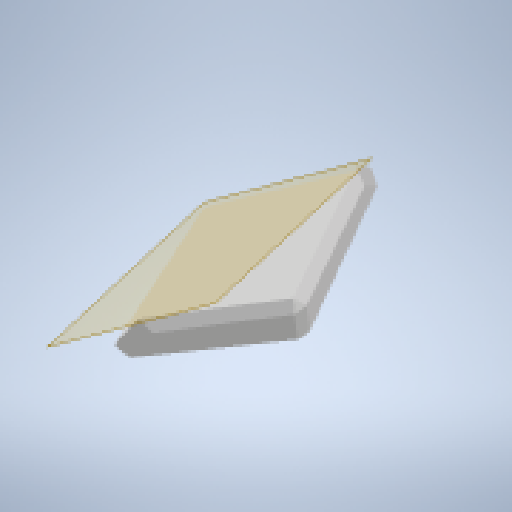
# Autodesk Inventor part: Union
Saved by Autodesk Inventor 2024 (Build 280153000, 153)
## iProperties
Created: 2024-04-21
Part Number: Union
Material: Genérico
Document SubType Name: Modeling
Designer: sergi
Density: 1 g/cm^3
Appearance: Valor por defecto
Author: sergi
Autodesk Inventor part; units mm, degrees
ref_plane "YZ Plane" through (0, 0, 0) normal (1, 0, 0) x (0, 1, 0)
ref_plane "XZ Plane" through (0, 0, 0) normal (0, 1, 0) x (-1, 0, 0)
ref_plane "XY Plane" through (0, 0, 0) normal (0, 0, 1) x (1, 0, 0)
ref_plane "Plano de trabajo1" through (154.464, -212.6015, -162.4131) normal (0.8506508, -0.2763932, -0.4472136) x (0.5, 0.688191, 0.5257311)
sketch "Boceto1" plane through (154.464, -212.6015, -162.4131) normal (0.8506508, -0.2763932, -0.4472136) x (0.5, 0.688191, 0.5257311)
  line L0 (7.992, -11) -> (13.5967, 0) projected
  line L1 (7.992, -11) -> (0, 0) projected
  line L2 (118, 0) -> (0, 0) projected
  line L3 (7.2654, -0.0037) -> (7.2604, -10.0037)
  line L4 (7.992, -11) -> (13.5967, 0)
  line L5 (7.2604, -10.0037) -> (13.3009, 1.8515)
  point P0 (154.464, -50.1884)
  point P1 (7.2636, -9.9974)
  point P2 (12.3575, 0)
  constraints: 6 end point, 1 collinear, 1 parallel, 3 other
extrude "Extrusión1" add sketch "Boceto1" along normal blind 1 contours L1 L2 L5
mirror "Simetría1" about plane through (154.464, -212.6015, -162.4131) normal (-0.5, -0.1624598, -0.8506508)
sketch "Boceto2" plane through (150.2624, -206.8184, -173.9792) normal (-0.4253254, -0.8618034, -0.2763932) x (0.8506508, -0.2763932, -0.4472136)
  line L0 (1, 1.2393) -> (1, 13.5967) projected
  line L1 (0, 13.5967) -> (1, 13.5967) projected
  line L2 (0, 1.2393) -> (0, 13.5967) projected
  line L3 (0, 13.5967) -> (1.5506, 14.6037)
  line L4 (0, 13.5967) -> (1.8488, 13.5967) construction
  line L5 (1, 13.5967) -> (1, 16)
  line L6 (1, 1.2393) -> (1, 13.5967) projected
  line L7 (0, 13.5967) -> (1, 13.5967) projected
  line L8 (0, 1.2393) -> (0, 13.5967) projected
  line L9 (0, 1.2393) -> (1, 1.2393) projected
  line L10 (0, 1.2393) -> (1, 1.2393) projected
  point P0 (-262.7899, 13.5967)
  point P1 (1, 14.2462)
  dimension "d8" = 33
  constraints: 6 end point, 1 equal length, 1 horizontal, 1 other
  measures "d8" angle of L4 L3
sketch3d "Boceto 3D1"
  line L0 (154.464, -212.6015, -162.4131) -> (161.2624, -203.2443, -155.2648)
sweep "Barrido1" add profiles "Boceto2" path "Boceto 3D1" contours L1 L3 L5
ref_plane "Plano de trabajo2" through (155.3147, -212.8779, -162.8603) normal (-0.5, -0.1624598, -0.8506508) x (0.1624598, 0.9472136, -0.2763932)
sketch "Boceto4" plane through (154.464, -212.6015, -162.4131) normal (-0.3087765, -0.4255001, 0.8506508) x (0.8091088, -0.5876588, -0.0002528)
  line L0 (0, 13.5967) -> (0.8508, 12.4744) projected
  line L1 (1.1754, 0.2007) -> (0, 0) projected
  line L2 (1.1754, 0.2007) -> (1.1754, 13.7974) projected
  line L3 (0, 13.5967) -> (1.1754, 13.7974) projected
  line L4 (0, 12.3575) -> (0, 0) projected
  line L5 (0.8508, 12.3575) -> (0.8508, 13.5967) projected
  line L6 (0.8508, 12.4744) -> (1.1754, 12.097)
  line L7 (0, 12.3575) -> (0, 13.5967) projected
  point P0 (-249.9564, 154.464)
  point P1 (0, 13.5967)
  constraints: 2 end point, 1 point on line
extrude "Extrusión2" cut sketch "Boceto4" against normal blind 1 contours L3 L2 L6 L0
mirror "Simetría2" about plane through (155.3147, -212.8779, -162.8603) normal (-0.5, -0.1624598, -0.8506508)
sketch "Boceto5" plane through (154.99, -213.3248, -163.2017) normal (0.1624598, -0.6708204, 0.7236068) x (0.8826329, 0.426631, 0.1973452)
  line L0 (0, 1.1924) -> (0.5446, 0.3537) projected
  line L1 (0, 0) -> (0, 1.1924) projected
  line L2 (0.5446, 0.3537) -> (0, 0) projected
  line L3 (0, 1.1924) -> (0.5446, 0.3537) projected
  line L4 (0.5446, 0.3537) -> (0.7129, 0.463) projected
  line L5 (0.7129, 0.463) -> (0, 1.1924) projected
  point P0 (-13.5812, 305.7136)
sketch3d "Boceto 3D2"
  line L0 (155.3147, -212.8779, -162.8603) -> (155.5153, -213.1541, -162.3079)
sweep "Barrido2" add profiles "Boceto5" path "Boceto 3D2" contours L0 L2 L1
ref_plane "Plano de trabajo3" through (161.3896, -204.5167, -155.8551) normal (-0.3087765, -0.4255001, 0.8506508) x (0.9468345, -0.0525626, 0.3173981)
split "Dividir1" plane through (161.3896, -204.5167, -155.8551) removes the side toward (-0.3087765, -0.4255001, 0.8506508)
sketch "Boceto6" plane through (161.4635, -204.9671, -156.0536) normal (0.9394777, 0.0031503, 0.3425955) x (0.3087765, 0.4255001, -0.8506508)
  line L0 (0, 0.4978) -> (0.5255, 0.4978) projected
  line L1 (0.5255, 0.4978) -> (0, 0) projected
  line L2 (0, 0.4978) -> (0.5255, 0.4978) projected
  line L3 (0, 0) -> (0, 0.4978) projected
  point P0 (-95.3897, 271.6858)
  point P1 (0, 0.4978)
sketch "Boceto7" plane through (155.3147, -212.8779, -162.8603) normal (0.8506508, -0.2763932, -0.4472136) x (-0.1624598, 0.6708204, -0.7236068)
  line L0 (0, 12.4744) -> (-0.6176, 12.097) projected
  line L1 (-0.6176, -0.4487) -> (-0.6176, 12.097) projected
  line L2 (11.3141, -4.3256) -> (-0.6176, -0.4487) projected
  line L3 (11.8639, -3.8548) -> (11.3141, -4.3256) projected
  line L4 (-0.6176, -0.4487) -> (-0.6176, -9.3178)
  line L5 (0, 12.3575) -> (0, 12.4744) projected
  line L6 (11.7527, -3.8187) -> (11.8639, -3.8548) projected
  line L7 (9.9974, 7.2636) -> (11.7527, -3.8187) projected
  line L8 (9.9974, 7.2636) -> (0, 12.3575) projected
  point P0 (50.1884, 154.464)
  constraints: 2 end point, 1 vertical
sweep "Barrido3" cut profiles "Boceto6" path "Boceto7" path curves L1 L4
mirror "Simetría6" about plane through (155.3147, -212.8779, -162.8603) normal (-0.5, -0.1624598, -0.8506508) of "Barrido3"
mirror "Simetría3" about plane through (154.464, -212.6015, -162.4131) normal (-0.3087765, -0.4255001, 0.8506508)
mirror "Simetría4" about plane through (154.464, -212.6015, -162.4131) normal (-0.5002052, -0.162646, -0.8504946)
ref_plane "Plano de trabajo6" through (150.8933, -207.6868, -150.2488) normal (-0.5261401, 0.7235753, -0.4467834) x (0.8398993, 0.3598484, -0.4062982)
sketch "Boceto9" plane through (150.8933, -207.6868, -150.2488) normal (-0.5261401, 0.7235753, -0.4467834) x (0.8398993, 0.3598484, -0.4062982)
  line L0 (-1.0032, 10.9782) -> (0.5612, 1.1013)
  line L1 (0.5612, 1.1013) -> (9.4712, 5.6413)
  line L2 (11.783, 1.1042) -> (6.1728, 12.1148) projected
  line L3 (-6.0326, 10.1817) -> (6.1728, 12.1148) projected
  line L4 (0.5626, 1.1042) -> (-6.0326, 10.1817) projected
  line L5 (0.5626, 1.1042) -> (11.783, 1.1042) projected
  point P0 (-113.0453, -221.9888)
  point P1 (0.5667, 1.1042)
  point P2 (9.4712, 5.6413)
  point P3 (-1.0032, 10.9782)
  point P4 (0.5602, 1.1075)
  constraints: 4 end point, 5 other
ref_plane "Plano de trabajo7" through (15.2836, -245.3662, -201.5907) normal (-0.3096114, 0.9508632, -0.0000964) x (-0.3620013, -0.1177778, 0.9247072)
extrude "Extrusión4" add sketch "Boceto9" along normal blind 15 contours L3 L2 L1 L0
ref_plane "Plano de trabajo9" through (40.3777, -55.7223, -51.0702) normal (0.3094977, -0.4249759, 0.8506507) x (0.2899736, 0.8941455, 0.3412025)
sketch "Boceto10" plane through (40.3777, -55.7223, -51.0702) normal (0.3094977, -0.4249759, 0.8506507) x (0.2899736, 0.8941455, 0.3412025)
  line L0 (-128.7402, -168) -> (-144, -168)
  line L1 (-144, -168) -> (-144, -153.0411)
  line L2 (-144, -153.0411) -> (-128.7402, -153.0411)
  line L3 (-128.7402, -153.0411) -> (-128.7402, -168)
  point P0 (55.5406, 64.8533)
  constraints: 8 end point, 2 parallel, 1 horizontal, 1 perpendicular
extrude "Extrusión5" cut sketch "Boceto10" against normal blind 10
sketch "Boceto11" plane through (151.2163, -208.1376, -151.3592) normal (-0.8087197, -0.2632746, 0.5259838) x (0.2629622, 0.6380637, 0.7236889)
  line L0 (0.0016, 7.8629) -> (-7.4458, 12.4595)
  point P0 (202.5779, 162.5394)
  constraints: 2 end point, 3 other
sketch "Boceto12" plane through (40.3777, -55.7223, -51.0702) normal (-0.3094977, 0.4249759, -0.8506507) x (-0.9056084, 0.1410648, 0.3999678)
  line L0 (-158.0595, -140.7536) -> (-163.7433, -134.0988)
  point P0 (64.8533, 55.5406)
  constraints: 2 end point, 3 other
ref_plane "Plano de trabajo12" through (149.7799, -198.7246, -162.3171) normal (0.5777995, -0.7943279, -0.1875926) x (-0.3085361, -0.4253622, 0.8508069)
split "Dividir2" plane through (149.7799, -198.7246, -162.3171) removes the side toward (-0.5777995, 0.7943279, 0.1875926)
sketch "Boceto13" plane through (150.6394, -207.3498, -172.925) normal (-0.8504577, 0.276456, 0.4475419) x (0.5195094, 0.5750731, 0.6319818)
  line L0 (4.582, -3.3803) -> (11.2177, 0.0007) projected
  line L1 (11.2243, 0.0041) -> (12.3837, -7.3498) projected
  line L2 (12.3798, -7.3535) -> (4.582, -3.3803) projected
  line L3 (11.2224, -0.0028) -> (5.6102, -11.0106) projected
  line L4 (12.7867, -9.8777) -> (5.6102, -11.0106) projected
  line L5 (17.8165, -9.0836) -> (12.7867, -9.8777) projected
  line L6 (11.2259, -0.0028) -> (17.8165, -9.0836) projected
  line L7 (11.2259, -0.0028) -> (11.2224, -0.0028) projected
  line L8 (11.2224, -0.0028) -> (5.6102, -11.0106) projected
  line L9 (11.2204, 0) -> (11.2224, -0.0028) projected
  line L10 (11.2204, 0) -> (0, 0) projected
  line L11 (0, 0) -> (5.6102, -11.0106) projected
  line L12 (11.2204, 0) -> (12.7867, -9.8777)
  line L13 (11.2204, 0) -> (1.5274, -4.9388)
  point P0 (150.2682, 62.6963)
  point P1 (5.6102, -11.0106)
  point P2 (2.3126, -4.5387)
  constraints: 4 end point, 1 perpendicular
extrude "Extrusión6" add sketch "Boceto13" along normal up to surface (7.8583 mm away) contours L0 L3 L2 | L2 L3 L11 L13 | L1 L12 L4 L3
sketch "Boceto14" plane through (142.7094, -210.9017, -165.8259) normal (-0.0004461, 0.8945091, 0.4470494) x (0.7074641, -0.3156695, 0.6323348)
  line L0 (-0.0028, -0.0014) -> (3.377, 6.6318) projected
  line L1 (7.3502, -1.166) -> (-0.0028, -0.0014) projected
  line L2 (11.8938, 5.4703) -> (9.9606, -6.735) projected
  line L3 (0, 11.2204) -> (4.5387, 8.9078) projected
  line L4 (0, 0) -> (0, 11.2204) projected
  line L5 (0, 0) -> (9.0775, -6.5952) projected
  line L6 (9.0775, -6.5952) -> (9.874, -1.5658) projected
  line L7 (9.874, -1.5658) -> (11.0106, 5.6102) projected
  line L8 (4.5387, 8.9078) -> (11.0106, 5.6102) projected
  line L9 (9.874, -1.5658) -> (-0.0028, -0.0014) projected
  line L10 (0, 0) -> (9.874, -1.5658)
  line L11 (4.5387, 8.9078) -> (1.3487, 2.647) projected
  line L12 (-0.0028, -0.0014) -> (3.4653, 6.8052) projected
  line L13 (-0.0028, -0.0014) -> (-0.0028, -0.0014) projected
  line L14 (-0.0028, -0.0056) -> (5.374, 10.5512)
  point P0 (-62.6795, -139.0149)
  point P1 (4.5373, 8.9085)
  constraints: 4 end point
extrude "Extrusión7" add sketch "Boceto14" along normal up to surface (7.857 mm away) contours L0 L11 L8 L7 L9 L1
ref_plane "Plano de trabajo13" through (150.6453, -207.3455, -172.925) normal (-0.0822425, 0.7702183, -0.6324555) x (0.8506508, -0.2763932, -0.4472136)
split "Dividir3" plane through (150.6453, -207.3455, -172.925) removes the side toward (-0.0822425, 0.7702183, -0.6324555)
ref_plane "Plano de trabajo14" through (150.6398, -208.2443, -173.372) normal (-0.7074641, 0.3156695, -0.6323348) x (-0.7067492, -0.3165535, 0.6326923)
split "Dividir4" plane through (150.6398, -208.2443, -173.372) removes the side toward (-0.7074641, 0.3156695, -0.6323348)
ref_plane "Plano de trabajo15" through (142.7098, -211.7962, -166.273) normal (-0.987609, -0.0705513, 0.1401817) x (0.1569337, -0.4414475, 0.8834568)
ref_plane "Plano de trabajo16" through (144.9964, -216.5785, -155.4664) normal (-0.6011922, 0.0550954, 0.7972029) x (0.601452, 0.6880431, 0.4060199)
ref_plane "Plano de trabajo17" through (151.7449, -208.8584, -150.9107) normal (0.133213, 0.5890228, 0.7970611) x (0.8398993, 0.3598484, -0.4062982)
ref_plane "Plano de trabajo18" through (160.645, -204.094, -155.9226) normal (0.371709, 0.9178244, 0.1393941) x (0.8504577, -0.276456, -0.4475419)
split "Dividir5" plane through (142.7098, -211.7962, -166.273) removes the side toward (-0.987609, -0.0705513, 0.1401817)
split "Dividir6" plane through (144.9964, -216.5785, -155.4664) removes the side toward (-0.6011922, 0.0550954, 0.7972029)
split "Dividir7" plane through (151.7449, -208.8584, -150.9107) removes the side toward (0.133213, 0.5890228, 0.7970611)
split "Dividir8" plane through (160.645, -204.094, -155.9226) removes the side toward (0.371709, 0.9178244, 0.1393941)
